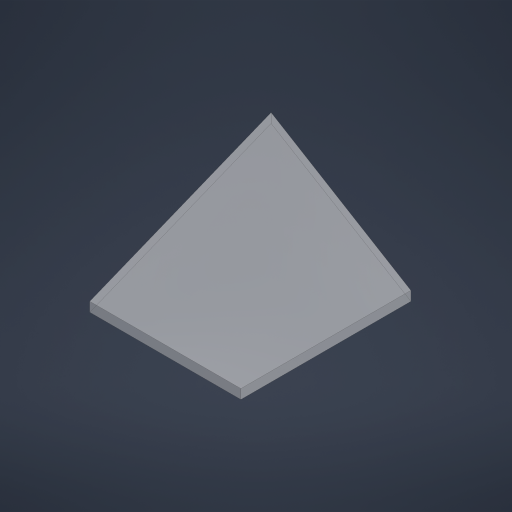
# Autodesk Inventor part: IntakeSleds
Saved by Autodesk Inventor 2024 (Build 280153000, 153)
## iProperties
Created: 2023-11-06
Part Number: IntakeSleds
Material: Polycarbonate, Clear
Document SubType Name: Sheet Metal
Designer: abhin
Density: 1.2 g/cm^3
Flat Pattern Width: 3.22917 cm
Flat Pattern Length: 5.14503 cm
Flat Pattern Area: 16.6142 cm^2
Sheet Metal Rule: Default
Sheet Metal Width: 1.271 in
Sheet Metal Length: 2.026 in
Sheet Metal Area: 2.575 in^2
Appearance: Polycarbonate - Clear
Author: abhin
Autodesk Inventor part; units mm, degrees
ref_plane "YZ Plane" through (0, 0, 0) normal (1, 0, 0) x (0, 1, 0)
ref_plane "XZ Plane" through (0, 0, 0) normal (0, 1, 0) x (-1, 0, 0)
ref_plane "XY Plane" through (0, 0, 0) normal (0, 0, 1) x (1, 0, 0)
sketch "Sketch1" plane through (0, 0, 0) normal (0, 1, 0) x (-1, 0, 0)
  line L0 (0, 0) -> (0, -28.575)
  line L1 (0, 0) -> (25.4, 0)
  line L2 (25.4, 0) -> (37.6506, -42.7285)
  line L3 (37.6506, -42.7285) -> (0, -28.575)
  dimension "d0" = 28.575
  dimension "d1" = 25.4
  dimension "d2" = 44.45
  constraints: 8 end point, 1 horizontal, 1 vertical
  measures "d0" distance of L0.start L0.end
  measures "d1" distance of L0.start L1.end
  measures "d2" distance of L1.end L2.end
extrude "Extrusion1" add sketch "Sketch1" along normal blind 1.5875
equation "\"BendRadius\" = Thickness"
equation "\"BendReliefWidth\" = Thickness"
equation "\"BendReliefDepth\" = 0.5 * Thickness"
equation "\"CornerReliefSize\" = 4 * Thickness"
equation "\"MinimumRemnant\" = 2 * Thickness"
equation "\"TransitionRadius\" = BendRadius"
equation "\"JacobiRadiusSize\" = BendRadius"
equation "\"GapSize\" = Thickness"
equation "\"Thickness\" = 1.5875"
body "Solid1"
